Buckle (Autodesk Fusion 360 design; units mm, degrees)
Autodesk Fusion 360 part; units mm, degrees
sketch "Sketch1" plane through (0, 0, 0) normal (0, 0, 1) x (1, 0, 0)
  line L0 (32.604, 29.4843) -> (52.304, 29.4843)
  line L1 (52.304, 29.4843) -> (52.304, 11.8843)
  line L2 (52.304, 11.8843) -> (32.604, 11.8843)
  line L3 (32.604, 11.8843) -> (32.604, 29.4843)
  line L4 (35.604, 26.4843) -> (49.304, 26.4843)
  line L5 (49.304, 26.4843) -> (49.304, 23.1843)
  line L6 (49.304, 23.1843) -> (35.604, 23.1843)
  line L7 (35.604, 23.1843) -> (35.604, 26.4843)
  line L8 (35.604, 18.1843) -> (49.304, 18.1843)
  line L9 (49.304, 18.1843) -> (49.304, 14.8843)
  line L10 (49.304, 14.8843) -> (35.604, 14.8843)
  line L11 (35.604, 14.8843) -> (35.604, 18.1843)
  dimension "d2" = 3.3
  dimension "d3" = 3.3
  dimension "d4" = 13.7
  dimension "d5" = 13.7
  dimension "d6" = 5
  dimension "d7" = 3
  dimension "d8" = 3
  dimension "d9" = 3
  dimension "d10" = 3
  dimension "d11" = 3
  constraint horizontal L0
  constraint vertical L1
  constraint horizontal L2
  constraint vertical L3
  constraint horizontal L4
  constraint vertical L5
  constraint horizontal L6
  constraint vertical L7
  constraint horizontal L8
  constraint vertical L9
  constraint horizontal L10
  constraint vertical L11
  measures "d2" distance of L8 L10
  measures "d3" distance of L4 L6
  measures "d4" distance of L4.start L4.end
  measures "d5" distance of L8.start L8.end
  measures "d6" distance of L6 L8
  measures "d7" distance of L0 L4
  measures "d8" distance of L2 L10
  measures "d9" distance of L3 L11
  measures "d10" distance of L3 L7
  measures "d11" distance of L1 L5
extrude "Extrude1" add sketch "Sketch1" along normal blind 3.5
fillet "Fillet1" radius 2.5 4 edges at (32.604, 29.4843, 1.75) (52.304, 29.4843, 1.75) (32.604, 11.8843, 1.75) (52.304, 11.8843, 1.75)
fillet "Fillet2" radius 0.5 16 edges at (51.5717, 12.6165, 3.5) (52.304, 20.6843, 3.5) (51.5717, 28.752, 3.5) (42.454, 29.4843, 3.5) (33.3362, 28.752, 3.5) (32.604, 20.6843, 3.5) (33.3362, 12.6165, 3.5) (42.454, 11.8843, 3.5) (33.3362, 12.6165, 0) (32.604, 20.6843, 0) (33.3362, 28.752, 0) (42.454, 29.4843, 0) (51.5717, 28.752, 0) (52.304, 20.6843, 0) (51.5717, 12.6165, 0) (42.454, 11.8843, 0)
equation "d3 = 3 mm + 0.3 mm"
equation "d4 = 0.5 in + 1 mm"
equation "d5 = 0.5 in + 1 mm"
